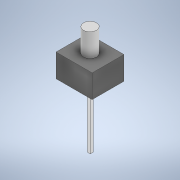
# Autodesk Inventor part: pata
Saved by Autodesk Inventor 2020 (Build 240168000, 168)
## iProperties
Created: 2021-10-19
Part Number: pata
Material: Genérico
Document SubType Name: Modeling
Designer: DANIEL
Density: 1 g/cm^3
Appearance: Valor por defecto
Author: DANIEL
Autodesk Inventor part; units mm, degrees
ref_plane "YZ Plane" through (0, 0, 0) normal (1, 0, 0) x (0, 1, 0)
ref_plane "XZ Plane" through (0, 0, 0) normal (0, 1, 0) x (-1, 0, 0)
ref_plane "XY Plane" through (0, 0, 0) normal (0, 0, 1) x (1, 0, 0)
sketch "Boceto1" plane through (0, 0, 0) normal (0, 1, 0) x (-1, 0, 0)
  line L0 (0.1, 0.1) -> (-0.1, 0.1)
  line L1 (-0.1, 0.1) -> (-0.1, -0.1)
  line L2 (-0.1, -0.1) -> (0.1, -0.1)
  line L3 (0.1, -0.1) -> (0.1, 0.1)
  point P0 (0, 0)
  dimension "L" = 0.2
  dimension "d1" = 0.2
  dimension "d2" = 0.1
  dimension "d3" = 0.1
  constraints: 8 end point, 2 parallel, 1 horizontal, 1 perpendicular
  measures "L" distance between parallel lines of L2 L0
  measures "d1" distance between parallel lines of L1 L3
  measures "d2" distance from line of L0 point (0, 0)
  measures "d3" distance from line of L3 point (0, 0)
extrude "Extrusión1" add sketch "Boceto1" along normal blind 11
sketch "Boceto2" plane through (0, 11, 0) normal (0, 1, 0) x (1, 0, 0)
  line L0 (-1.183, 1.017) -> (1.317, 1.017)
  line L1 (1.317, 1.017) -> (1.317, -1.183)
  line L2 (1.317, -1.183) -> (-1.183, -1.183)
  line L3 (-1.183, -1.183) -> (-1.183, 1.017)
  point P0 (0, 0)
  dimension "d6" = 2.2
  dimension "d7" = 2.5
  constraints: 8 end point, 2 parallel, 1 horizontal, 1 perpendicular
  measures "d6" distance between parallel lines of L2 L0
  measures "d7" distance between parallel lines of L1 L3
extrude "Extrusión2" add sketch "Boceto2" against normal blind 1.6
ref_plane "Plano de trabajo1" through (0.067, 11, 1.183) normal (1, 0, 0) x (0, 0, -1)
ref_plane "Plano de trabajo2" through (-1.183, 11, 0.083) normal (0, 0, 1) x (1, 0, 0)
ref_plane "Plano de trabajo3" through (-1.183, 11, 0.083) normal (0, 0, 1) x (1, 0, 0)
ref_plane "Plano de trabajo4" through (0, 11, 0) normal (0, 1, 0) x (1, 0, 0)
sketch "Boceto3" plane through (0, 11, 0) normal (0, 1, 0) x (1, 0, 0)
  circle A0 centre (0.067, -0.083) radius 0.45
  line L0 (1.317, -1.183) -> (1.317, 1.017) projected
  line L1 (1.317, 1.017) -> (-1.183, 1.017) projected
  line L2 (-1.183, 1.017) -> (-1.183, -1.183) projected
  line L3 (-1.183, -1.183) -> (1.317, -1.183) projected
  point P0 (0, 0)
  dimension "d11" = 0.9
  dimension "d12" = 1.1
  dimension "d13" = 1.25
  constraints: 1 centre point
  measures "d11" diameter of A0
  measures "d12" distance from line of L1 A0.centre
  measures "d13" distance from line of A0.centre L2
extrude "Extrusión3" add sketch "Boceto3" along normal blind 1.6 contours A0
sketch "Boceto4" plane through (0, 0, 0) normal (0, -1, 0) x (1, 0, 0)
  line L0 (0.1, 0.1) -> (0.1, -0.1) projected
  line L1 (-0.1, 0.1) -> (0.1, 0.1) projected
  line L2 (-0.1, -0.1) -> (-0.1, 0.1) projected
  line L3 (0.1, -0.1) -> (-0.1, -0.1) projected
  line L4 (0.1, -0.1) -> (0.1, 0.1) projected
  line L5 (0.1, 0.1) -> (-0.1, 0.1)
  line L6 (-0.1, 0.1) -> (-0.1, -0.1)
  line L7 (-0.1, -0.1) -> (0.1, -0.1)
  line L8 (0.1, -0.1) -> (0.1, 0.1)
  point P0 (0, 0)
  constraints: 8 end point, 2 parallel, 1 horizontal, 1 perpendicular
extrude "Extrusión4" cut sketch "Boceto4" against normal blind 5
equation "\"d1\" = L"
equation "\"d2\" = 0.5 * L"
equation "\"d3\" = 0.5 * L"
